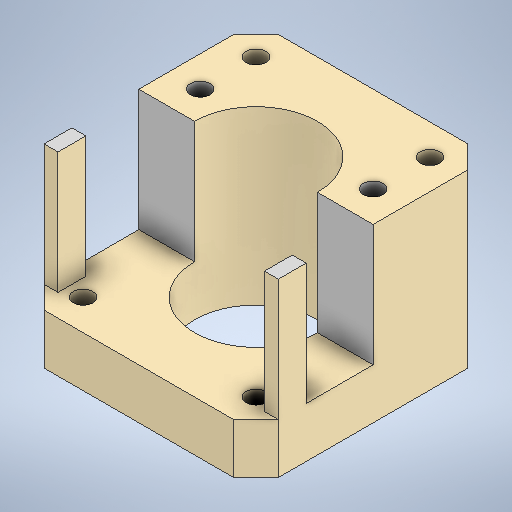
# Autodesk Inventor part: Base for NEMA17
Saved by Autodesk Inventor 2025 (Build 290162000, 162)
## iProperties
Created: 2025-07-19
Part Number: Base for NEMA17
Material: Generic
Document SubType Name: Modeling
Designer: yshis
Density: 1 g/cm^3
Appearance: Default
Author: yshis
Autodesk Inventor part; units mm, degrees
ref_plane "YZ Plane" through (0, 0, 0) normal (1, 0, 0) x (0, 1, 0)
ref_plane "XZ Plane" through (0, 0, 0) normal (0, 1, 0) x (-1, 0, 0)
ref_plane "XY Plane" through (0, 0, 0) normal (0, 0, 1) x (1, 0, 0)
sketch "Sketch1" plane through (0, 0, 0) normal (0, 1, 0) x (-1, 0, 0)
  line L0 (0, 0) -> (42, 0)
  line L1 (42, 0) -> (42, -42)
  line L2 (42, -42) -> (0, -42)
  line L3 (0, -42) -> (0, 0)
  circle A0 centre (5.5, -5.5) radius 1.75
  circle A1 centre (5.5, -36.5) radius 1.75
  circle A2 centre (36.5, -5.5) radius 1.75
  circle A3 centre (36.5, -36.5) radius 1.75
  circle A4 centre (21, -21) radius 11
  point P0 (0, -31)
  point P1 (31, 0)
  point P2 (31, -31)
  dimension "d0" = 42
  dimension "d1" = 42
  dimension "d2" = 3.5
  dimension "d5" = 31
  dimension "d8" = 31
  dimension "d11" = 5.5
  dimension "d12" = 5.5
  dimension "d13" = 22
  constraints: 8 end point, 5 centre point, 2 horizontal, 2 parallel, 1 perpendicular, 1 vertical, 9 other
  measures "d0" distance of L1.end L2.end
  measures "d1" distance of L0.end L1.end
  measures "d2" diameter of A0
  measures "d5" distance of L0.start point (0, -31)
  measures "d8" distance of L0.start point (31, 0)
  measures "d11" horizontal distance of A0.centre L0.start
  measures "d12" horizontal distance of L0.start A0.centre
  measures "d13" diameter of A4
extrude "Extrusion1" add sketch "Sketch1" along normal blind 9
sketch "Sketch2" plane through (0, 9, 0) normal (0, 1, 0) x (1, 0, 0)
  line L0 (0, 42) -> (-42, 42) projected
  line L1 (-42, 4) -> (-42, 42)
  line L2 (-42, 42) -> (0, 42)
  line L3 (0, 42) -> (0, 4)
  circle A0 centre (-21, 21) radius 11 projected
  arc A1 (-10, 21) -> (-32, 21) centre (-21, 21) ccw
  line L4 (-42, 0) -> (0, 0) projected
  line L5 (-39.5, 9) -> (-39.5, 4)
  line L6 (-39.5, 4) -> (-42, 4)
  line L7 (-2.5, 9) -> (-2.5, 4)
  line L8 (-2.5, 4) -> (0, 4)
  circle A2 centre (-36.5, 36.5) radius 1.75 projected
  circle A3 centre (-36.5, 36.5) radius 1.75
  circle A4 centre (-5.3062, 36.5) radius 1.7607
  line L9 (0, 0) -> (-32, 0)
  line L10 (-39.5, 0) -> (-42, 0)
  line L11 (-2.5, 9) -> (0, 9)
  line L12 (-39.5, 9) -> (-42, 9)
  line L13 (-42, 42) -> (-42, 0) projected
  line L14 (-32, 21) -> (-42, 21)
  line L15 (-10, 21) -> (0, 21)
  point P0 (-42, 12)
  point P1 (0, 12)
  dimension "d19" = 4
  dimension "d20" = 2.5
  dimension "d25" = 2.5
  dimension "d34" = 5
  dimension "d36" = 5
  dimension "d37" = 4
  constraints: 26 end point, 7 point on line, 6 perpendicular, 3 centre point, 3 parallel, 2 coincident, 2 horizontal, 2 point on circle, 2 vertical, 1 midpoint
  measures "d19" distance of L1.start L4.start
  measures "d20" distance between parallel lines of L1 L5
  measures "d25" distance between parallel lines of L7 L3
  measures "d34" distance between parallel lines of L12 L6
  measures "d36" distance between parallel lines of L11 L8
  measures "d37" distance between parallel lines of L8 L9
chamfer "Chamfer1" distance 4 angle 45 4 edges at (0, 4.5, -42) (-42, 4.5, -42) (-42, 4.5, 0) (0, 4.5, 0)
extrude "Extrusion2" add sketch "Sketch2" along normal blind 21.8 contours L3 L15 A0 L14 L1 L0 | L1 L12 L5 L6 | L3 L8 L7 L11
chamfer "Chamfer5" distance 4 angle 45 1 edges at (-42, 19.9, -42)
chamfer "Chamfer6" distance 4 angle 45 1 edges at (0, 19.9, -42)
sketch "Sketch3" plane through (0, 30.8, 0) normal (0, 1, 0) x (1, 0, 0)
  circle A0 centre (-36.5, 26.5) radius 1.75
  circle A1 centre (-36.5, 36.5) radius 1.75 projected
  circle A2 centre (-5.5, 26.5) radius 1.75
  circle A3 centre (-5.3062, 36.5) radius 1.7607 projected
  point P0 (0, 0)
  dimension "d48" = 3.5
  dimension "d49" = 10
  dimension "d50" = 3.5
  dimension "d51" = 10
  constraints: 2 centre point
  measures "d48" diameter of A0
  measures "d49" distance of A0.centre A1.centre
  measures "d50" diameter of A2
  measures "d51" vertical distance of A2.centre A3.centre
extrude "Extrusion3" cut sketch "Sketch3" against normal blind 30.8 contours A0 | A2
sketch "Sketch4" plane through (0, 0, 0) normal (0, -1, 0) x (1, 0, 0)
  circle A0 centre (-5.5, -26.5) radius 1.75 projected
  line L0 (-3.85, -29.3579) -> (-7.15, -29.3579)
  line L1 (-7.15, -29.3579) -> (-8.8, -26.5)
  line L2 (-8.8, -26.5) -> (-7.15, -23.6421)
  line L3 (-7.15, -23.6421) -> (-3.85, -23.6421)
  line L4 (-3.85, -23.6421) -> (-2.2, -26.5)
  line L5 (-2.2, -26.5) -> (-3.85, -29.3579)
  line L6 (-4, -42) -> (-38, -42) projected
  line L7 (-34.85, -29.3579) -> (-38.15, -29.3579)
  line L8 (-38.15, -29.3579) -> (-39.8, -26.5)
  line L9 (-39.8, -26.5) -> (-38.15, -23.6421)
  line L10 (-38.15, -23.6421) -> (-34.85, -23.6421)
  line L11 (-34.85, -23.6421) -> (-33.2, -26.5)
  line L12 (-33.2, -26.5) -> (-34.85, -29.3579)
  point P0 (0, 0)
  point P1 (-36.5, -26.5)
  point P2 (-36.5, -26.5)
  dimension "d55" = 5.7158
  dimension "d56" = 0
  dimension "d59" = 31
  constraints: 24 end point, 2 coincident, 1 horizontal, 27 other
  measures "d55" distance between parallel lines of L2 L5
  measures "d56" angle of L6 L0
  measures "d59" distance of A0.centre point (-36.5, -26.5)
extrude "Extrusion4" cut sketch "Sketch4" against normal blind 24.8 contours A0 | L0 L1 L2 L3 L4 L5 | L7 L8 L9 L10 L11 L12
equation "\"d11\" = -0.5 * d5 + 0.5 * d1"
equation "\"d12\" = d11"
equation "\"d25\" = d20"
equation "\"d36\" = d34"
equation "\"d37\" = d19"
equation "\"d51\" = d49"
equation "\"d23\" = d19"
equation "\"d24\" = d22"
equation "\"d22\" = 12"
body "Solid1"
